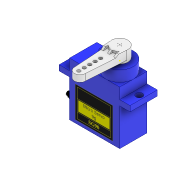
# Autodesk Inventor part: servo
Saved by Autodesk Inventor 2022 (Build 260153000, 153)
## iProperties
Created: 2022-11-16
Part Number: servo
Material: Generic
Document SubType Name: Modeling
Designer: ferna
Density: 1 g/cm^3
Appearance: Default
Author: ferna
Autodesk Inventor part; units mm, degrees
sketch "Sketch1" plane through (0, 0, 0) normal (0, 1, 0) x (-1, 0, 0)
  line L0 (0, 0) -> (23, 0)
  line L1 (23, 0) -> (23, -12.5)
  line L2 (23, -12.5) -> (0, -12.5)
  line L3 (0, -12.5) -> (0, 0)
  dimension "d0" = 23
  dimension "d1" = 12.5
  constraints: 8 end point, 2 parallel, 1 horizontal, 1 perpendicular
  measures "d0" distance of L1.end L2.end
  measures "d1" distance of L0.end L1.end
extrude "Extrusion1" add sketch "Sketch1" along normal blind 17
sketch "Sketch2" plane through (0, 17, 0) normal (0, 1, 0) x (1, 0, 0)
  line L0 (0, 0) -> (0, 12.5) projected
  line L1 (0, 0) -> (-11.5, 0)
  line L2 (-23, 12.5) -> (-23, 0) projected
  line L3 (-11.5, 0) -> (-11.5, 6.25)
  line L4 (-27.75, 0) -> (4.75, 0)
  line L5 (4.75, 0) -> (4.75, 12.5)
  line L6 (4.75, 12.5) -> (-27.75, 12.5)
  line L7 (-27.75, 12.5) -> (-27.75, 0)
  line L8 (-27.75, 0) -> (4.75, 12.5) construction
  line L9 (4.75, 0) -> (-27.75, 12.5) construction
  dimension "d4" = 11.5
  dimension "d5" = 6.25
  dimension "d6" = 32.5
  constraints: 16 end point, 3 perpendicular, 2 midpoint, 2 parallel, 1 horizontal
  measures "d4" distance of L0.start L1.end
  measures "d5" distance of L1.end L3.end
  measures "d6" distance of L6.end L5.end
extrude "Extrusion2" add sketch "Sketch2" along normal blind 2.5
sketch "Sketch3" plane through (0, 19.5, 0) normal (0, 1, 0) x (1, 0, 0)
  line L0 (0, 12.5) -> (-23, 12.5) projected
  line L1 (0, 0) -> (-23, 0)
  line L2 (-23, 0) -> (-23, 12.5)
  line L3 (-23, 12.5) -> (0, 12.5)
  line L4 (0, 12.5) -> (0, 0)
  constraints: 8 end point, 2 parallel, 1 horizontal, 1 perpendicular
extrude "Extrusion3" add sketch "Sketch3" along normal blind 5
sketch "Sketch4" plane through (0, 19.5, 0) normal (0, 1, 0) x (1, 0, 0)
  line L0 (4.75, 0) -> (4.75, 12.5) projected
  line L1 (4.75, 6.25) -> (2.75, 6.25)
  line L2 (-27.75, 12.5) -> (-27.75, 0) projected
  line L3 (-27.75, 6.25) -> (-25.75, 6.25)
  circle A0 centre (-25.75, 6.25) radius 1.5
  circle A1 centre (2.75, 6.25) radius 1.5
  point P0 (0, 0)
  dimension "d11" = 2
  dimension "d12" = 2
  dimension "d13" = 3
  dimension "d14" = 3
  constraints: 4 end point, 2 centre point, 2 coincident, 2 horizontal, 2 midpoint
  measures "d11" distance of L1.start L1.end
  measures "d12" distance of L3.start L3.end
  measures "d13" diameter of A0
  measures "d14" diameter of A1
extrude "Extrusion4" cut sketch "Sketch4" against normal blind 5
sketch "Sketch5" plane through (0, 24.5, 0) normal (0, 1, 0) x (1, 0, 0)
  line L0 (0, 0) -> (0, 12.5) projected
  line L1 (0, 6.25) -> (-6.25, 6.25)
  circle A0 centre (-6.25, 6.25) radius 6.25
  circle A1 centre (-12.5, 6.25) radius 2.5
  line L2 (-12.5, 8.75) -> (-11.9782, 8.75)
  line L3 (-12.5, 3.75) -> (-11.9782, 3.75)
  dimension "d17" = 6.25
  dimension "d20" = 5
  constraints: 6 end point, 6 point on circle, 2 centre point, 2 horizontal, 2 tangent, 1 coincident, 1 midpoint, 1 parallel
  measures "d17" distance of L1.start L1.end
  measures "d20" diameter of A1
extrude "Extrusion5" add sketch "Sketch5" along normal blind 5
sketch "Sketch7" plane through (0, 29.5, 0) normal (0, 1, 0) x (1, 0, 0)
  arc A0 (-11.9782, 3.75) -> (-11.9782, 8.75) centre (-6.25, 6.25) ccw projected
  circle A1 centre (-6.25, 6.25) radius 2.5
  point P0 (0, 0)
  dimension "d21" = 5
  constraints: 1 centre point, 1 coincident
  measures "d21" diameter of A1
extrude "Extrusion6" add sketch "Sketch7" along normal blind 0.5
sketch "Sketch8" plane through (-6.25, 30, -6.25) normal (0, 1, 0) x (1, 0, 0)
  circle A0 centre (0, 0) radius 3.75
  point P0 (6.25, -6.25)
  dimension "d24" = 7.5
  constraints: 1 centre point
  measures "d24" diameter of A0
extrude "Extrusion7" add sketch "Sketch8" along normal blind 5
ref_plane "Work Plane1" through (-6.25, 34, -6.25) normal (0, 1, 0) x (1, 0, 0)
sketch "Sketch9" plane through (-6.25, 34, -6.25) normal (0, 1, 0) x (1, 0, 0)
  circle A0 centre (0, 0) radius 3.75 projected
  line L0 (0, 3.75) -> (0, -18.25)
  circle A1 centre (0, -18.25) radius 2.5
  line L1 (-2.5, -18.25) -> (-3.75, 0)
  line L2 (2.5, -18.25) -> (3.75, 0)
  line L3 (-3.75, 0) -> (3.75, 0)
  line L4 (0, -20.75) -> (0, -18.75)
  line L5 (0, -18.75) -> (0, -16.25)
  line L6 (0, -16.25) -> (0, -13.75)
  line L7 (0, -13.75) -> (0, -11.25)
  line L8 (0, -11.25) -> (0, -8.75)
  circle A2 centre (0, -18.75) radius 0.75
  circle A3 centre (0, -16.25) radius 0.75
  circle A4 centre (0, -13.75) radius 0.75
  circle A5 centre (0, -11.25) radius 0.75
  circle A6 centre (0, -8.75) radius 0.75
  point P0 (6.25, -6.25)
  point P1 (3.715, -0.5113)
  point P2 (-3.715, -0.5113)
  dimension "d28" = 22
  dimension "d29" = 5
  dimension "d30" = 2
  dimension "d31" = 2.5
  dimension "d32" = 2.5
  dimension "d33" = 2.5
  dimension "d34" = 2.5
  dimension "d35" = 1.5
  dimension "d36" = 1.5
  dimension "d37" = 1.5
  dimension "d38" = 1.5
  dimension "d39" = 1.5
  constraints: 18 end point, 6 centre point, 6 coincident, 6 point on circle, 4 point on line, 1 horizontal, 1 perpendicular, 1 vertical
  measures "d28" distance of L0.start L0.end
  measures "d29" diameter of A1
  measures "d30" distance of L4.start L4.end
  measures "d31" distance of L4.end L5.end
  measures "d32" distance of L5.end L6.end
  measures "d33" distance of L6.end L7.end
  measures "d34" distance of L7.end L8.end
  measures "d35" diameter of A2
  measures "d36" diameter of A3
  measures "d37" diameter of A4
  measures "d38" diameter of A5
  measures "d39" diameter of A6
extrude "Extrusion8" add sketch "Sketch9" against normal blind 3 contours L2 A1 A3 L0 A4 A5 A6 A0 | L0 A6 A5 A4 A3 A1 L1 A0 | A1 L4 A2 L0 A3 | A1 A3 L0 A2 L4
sketch "Sketch10" plane through (-3.75, 31, 12) normal (0.9976626, 0, 0.0683331) x (0.0683331, 0, -0.9976626)
  line L0 (17.7803, 3) -> (14.2865, 3) projected
  line L1 (17.7803, 3) -> (17.7803, 4)
  line L2 (21.7865, 4) -> (14.2865, 4) projected
  line L3 (17.7803, 4) -> (14.2803, 4)
  line L4 (14.2803, 4) -> (13.0477, 3)
  line L5 (0, 3) -> (17.7803, 3) projected
  line L6 (17.7803, 3) -> (17.7803, 0) projected
  line L7 (13.0477, 3) -> (17.7803, 3)
  point P0 (12.2282, -31)
  point P1 (17.2725, 3)
  point P2 (14.2865, 4)
  dimension "d42" = 3.5
  dimension "d45" = 4.7325
  constraints: 8 end point, 2 point on line, 1 horizontal, 1 perpendicular, 1 vertical
  measures "d42" distance of L1.end L3.end
  measures "d45" distance of L0.start L4.end
extrude "Extrusion9" add sketch "Sketch10" against normal blind 1
sketch "Sketch12" plane through (-9.965, 31, -5.7387) normal (-0.9976626, 0, 0.0683331) x (0.0683331, 0, 0.9976626)
  line L0 (0, 0) -> (0, 3) projected
  line L1 (0, 3) -> (0, 4)
  line L2 (3.4938, 4) -> (-4.0062, 4) projected
  line L3 (0, 4) -> (3.5, 4)
  line L4 (0, 3) -> (4.733, 3)
  line L5 (0.5077, 0) -> (18.1219, 0) projected
  line L6 (0, 3) -> (4.733, 3) construction
  line L7 (3.5, 4) -> (4.733, 3)
  point P0 (6.4062, -31)
  point P1 (0.5077, 4)
  point P2 (2.6525, 4)
  point P3 (4.733, 3)
  dimension "d46" = 3.5
  dimension "d47" = 4.733
  dimension "d48" = 0
  constraints: 10 end point, 1 collinear, 1 horizontal, 1 parallel, 1 perpendicular, 1 point on line, 1 vertical
  measures "d46" distance of L1.end L3.end
  measures "d47" distance of L0.end L4.end
  measures "d48" distance between parallel lines of L6 L4
extrude "Extrusion10" add sketch "Sketch12" against normal blind 1
sketch "Sketch13" plane through (-6.25, 35, -6.25) normal (0, 1, 0) x (1, 0, 0)
  point P0 (6.25, -6.25)
  point P1 (0, 0)
ref_plane "Work Plane2" through (-6.25, 35, -6.25) normal (1, 0, 0) x (0, 0, -1)
sketch "Sketch14" plane through (-6.25, 35, -6.25) normal (1, 0, 0) x (0, 0, -1)
  line L0 (-3.9348, 0) -> (-5.1649, -1) projected
  line L1 (-5.1644, -1) -> (-3.9348, 0) projected
  line L2 (-2.7403, 0) -> (-3.75, 0) projected
  line L3 (-3.9348, 0) -> (-3.75, 0)
  line L4 (-2.7403, -1) -> (-3.75, -1) projected
  line L5 (-3.75, 0) -> (-3.75, -1)
  line L6 (-3.75, -1) -> (-5.1644, -1)
  line L7 (-3.75, 0) -> (-3.3986, 0)
  line L8 (-3.3986, 0) -> (-3.3986, -1)
  line L9 (-3.3986, -1) -> (-3.75, -1)
  line L10 (-3.75, -1) -> (-3.75, 0)
  point P0 (-6.25, -35)
  constraints: 14 end point, 3 perpendicular, 2 horizontal, 2 parallel, 1 point on line
extrude "Extrusion11" add sketch "Sketch14" along normal mid plane 1
sketch "Sketch15" plane through (-6.25, 35, -6.25) normal (1, 0, 0) x (0, 0, -1)
  line L0 (6.25, -5.5) -> (-6.25, -5.5) projected
  line L1 (6.25, -5.5) -> (-23.4835, -5.5)
  line L2 (-23.4835, -5.5) -> (-23.4835, 1.9861)
  line L3 (-23.4835, 1.9861) -> (6.25, 1.9861)
  line L4 (6.25, 1.9861) -> (6.25, -5.5)
  point P0 (-6.25, -35)
  point P1 (-2.5, -5.5)
  point P2 (2.5, -5.5)
  constraints: 8 end point, 2 parallel, 1 horizontal, 1 perpendicular
split body "Split1" sketch "Sketch15" result two bodies curves L4 L1 L2 L3 first body at (-7.6667, 5.6667, -12)
sketch "Sketch16" plane through (0, 0, -12.5) normal (0, 0, -1) x (-1, 0, 0)
  line L0 (2.4918, 15.6301) -> (19.8733, 15.6301) construction
  line L1 (19.8733, 15.6301) -> (19.8733, 1.2979) construction
  line L2 (19.8733, 1.2979) -> (2.4918, 1.2979) construction
  line L3 (2.4918, 1.2979) -> (2.4918, 15.6301) construction
  point P0 (0, 0)
  constraints: 2 other
decal "Decal1"
sketch "Sketch17" plane through (-23, 0, 0) normal (0, 0, 1) x (1, 0, 0)
  line L0 (2.4918, 15.6301) -> (19.8733, 15.6301) construction
  line L1 (19.8733, 15.6301) -> (19.8733, 1.2979) construction
  line L2 (19.8733, 1.2979) -> (2.4918, 1.2979) construction
  line L3 (2.4918, 1.2979) -> (2.4918, 15.6301) construction
  point P0 (23, 0)
  point P1 (0, 0)
  constraints: 2 other
decal "Decal2"
sketch "Sketch18" plane through (-23, 0, -12.5) normal (-1, 0, 0) x (0, 0, 1)
  line L0 (12.5, 0) -> (0, 0) projected
  line L1 (0, 0) -> (6.25, 0)
  line L2 (6.25, 0) -> (6.25, 4)
  circle A0 centre (6.25, 4) radius 0.65
  line L3 (6.9, 4) -> (7.55, 4)
  line L4 (5.6, 4) -> (4.95, 4)
  circle A1 centre (4.95, 4) radius 0.65
  circle A2 centre (7.55, 4) radius 0.65
  dimension "d67" = 6.25
  dimension "d68" = 4
  dimension "d69" = 1.3
  dimension "d70" = 0.65
  dimension "d71" = 0.65
  constraints: 8 end point, 3 coincident, 2 horizontal, 2 horizontal alignment, 2 point on circle, 1 centre point, 1 midpoint, 1 perpendicular, 4 other
  measures "d67" distance of L0.end L1.end
  measures "d68" distance of L1.end L2.end
  measures "d69" diameter of A0
  measures "d70" distance of L3.start L3.end
  measures "d71" distance of L4.start L4.end
extrude "Extrusion12" add sketch "Sketch18" along normal blind 3 bodies 2
sketch "Sketch19" plane through (-26, 4, -4.95) normal (-1, 0, 0) x (0, 0, 1)
  arc A0 (-0.65, 0) -> (-1.95, 0) centre (-1.3, 0) ccw projected
  arc A1 (-1.95, 0) -> (-0.65, 0) centre (-1.3, 0) ccw projected
  ellipse E0 centre (-1.3, 0) end of major axis (-1.3, 0.9472) minor radius 2.1084
  point P0 (4.95, -4)
  constraints: 1 coincident, 2 other
extrude "Extrusion13" add sketch "Sketch19" along normal blind 1 separate body contours A1 A0 | E0
ref_plane "Work Plane3" through (-30, 4, -4.95) normal (-1, 0, 0) x (0, 0, 1)
sketch "Sketch20" plane through (-30, 4, -4.95) normal (-1, 0, 0) x (0, 0, 1)
  arc A0 (-0.65, 0) -> (-1.95, 0) centre (-1.3, 0) ccw projected
  circle A1 centre (-1.3, 0) radius 0.94
  point P0 (4.95, -4)
  dimension "d77" = 1.88
  constraints: 1 centre point, 1 coincident
  measures "d77" diameter of A1
loft "Loft1" add profiles "Sketch20" bodies 4 section 1 edges at (-27, 4, -4.1416)
sketch "Sketch21" plane through (-30, 4, -6.25) normal (-1, 0, 0) x (0, 0, 1)
  circle A0 centre (0, 0) radius 0.94 projected
  point P0 (0.94, 0)
  constraints: 1 horizontal alignment
body "Solid4"
body "Solid2"
body "Solid3"
